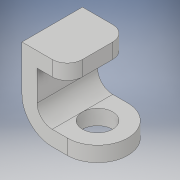
# Autodesk Inventor part: 零件18
Saved by Autodesk Inventor 2019 (Build 230136000, 136)
## iProperties
Created: 2020-09-18
Part Number: 零件18
Material: 一般
Document SubType Name: Modeling
Designer: jay
Density: 1 g/cm^3
Appearance: 預設
Author: jay
Autodesk Inventor part; units mm, degrees
ref_plane "YZ Plane" through (0, 0, 0) normal (1, 0, 0) x (0, 1, 0)
ref_plane "XZ Plane" through (0, 0, 0) normal (0, 1, 0) x (-1, 0, 0)
ref_plane "XY Plane" through (0, 0, 0) normal (0, 0, 1) x (1, 0, 0)
sketch "草圖1" plane through (0, 0, 0) normal (0, 0, 1) x (1, 0, 0)
  line L0 (0, 0) -> (50, 0)
  line L1 (50, 10) -> (10, 10)
  line L2 (10, 10) -> (10, 40)
  line L3 (10, 40) -> (30, 40)
  line L4 (30, 40) -> (30, 50)
  line L5 (30, 50) -> (0, 50)
  line L6 (0, 50) -> (0, 0)
  line L7 (50, 10) -> (50, 0)
  dimension "d0" = 50
  dimension "d1" = 10
  dimension "d2" = 30
  dimension "d3" = 30
  dimension "d4" = 10
  dimension "d5" = 50
  constraints: 16 end point, 5 perpendicular, 1 horizontal
  measures "d0" distance of L5.end L0.start
  measures "d1" distance of L0.end L1.start
  measures "d2" distance of L1.end L2.end
  measures "d3" distance of L4.end L5.end
  measures "d4" distance between parallel lines of L6 L2
  measures "d5" distance between parallel lines of L6 L7
extrude "擠出1" add sketch "草圖1" along normal mid plane 40
fillet "圓角1" radius 20 2 edges at (50, 5, 20) (50, 5, -20)
fillet "圓角2" radius 20 1 edges at (0, 0, 0)
fillet "圓角3" radius 10 1 edges at (10, 10, 0)
fillet "圓角4" radius 10 2 edges at (30, 45, 20) (30, 45, -20)
sketch "草圖2" plane through (30, 10, 0) normal (0, 1, 0) x (1, 0, 0)
  arc A0 (0, -20) -> (0, 20) centre (0, 0) ccw projected
  point P0 (-30, 0)
  constraints: 1 coincident
hole "孔1" at (30, 10, 0) direction (0, -1, 0) diameter 20 end through all
